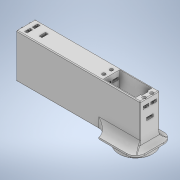
# Autodesk Inventor part: мотор_плеча_2.1-локтя_1_v2_увелич
Saved by Autodesk Inventor 2022 (Build 260153000, 153)
## iProperties
Created: 2022-12-03
Part Number: мотор_плеча_2.1-локтя_1_v2_увелич
Material: Типовые
Document SubType Name: Modeling
Designer: Папа
Density: 1 g/cm^3
Appearance: По умолчанию
Author: Папа
Autodesk Inventor part; units mm, degrees
(part 1 of 2)
ref_plane "YZ Plane" through (0, 0, 0) normal (1, 0, 0) x (0, 1, 0)
ref_plane "XZ Plane" through (0, 0, 0) normal (0, 1, 0) x (-1, 0, 0)
ref_plane "XY Plane" through (0, 0, 0) normal (0, 0, 1) x (1, 0, 0)
sketch "Эскиз1" plane through (0, 0, 0) normal (0, 1, 0) x (-1, 0, 0)
  line L0 (0, 0) -> (-59.05, 0)
  line L1 (-59.05, 0) -> (-59.05, -29.25)
  line L2 (-59.05, -29.25) -> (0, -29.25)
  line L3 (0, -29.25) -> (0, 0)
  line L4 (-74.05, 3) -> (15, 3)
  line L5 (15, 3) -> (15, -32.25)
  line L6 (15, -32.25) -> (-74.05, -32.25)
  line L7 (-74.05, -32.25) -> (-74.05, 3)
  line L8 (-74.05, 3) -> (15, -32.25) construction
  line L9 (15, 3) -> (-74.05, -32.25) construction
  line L10 (0, -29.25) -> (-59.05, 0) construction
  line L11 (0, 0) -> (-59.05, -29.25) construction
  line L12 (15, 0) -> (-74.05, 0)
  point P0 (-29.525, -14.625)
  point P1 (-29.525, -14.625)
  point P2 (-59.05, 0)
  point P3 (-59.05, 0)
  point P4 (0, 0)
  dimension "d0" = 29.25
  dimension "d1" = 59.05
  dimension "d2" = 15
  dimension "d3" = 3
  constraints: 26 end point, 4 midpoint, 4 parallel, 3 point on line, 2 horizontal, 2 perpendicular, 1 collinear
  measures "d0" distance of L2.end L0.start
  measures "d1" distance of L1.end L2.end
  measures "d2" distance between parallel lines of L3 L5
  measures "d3" distance between parallel lines of L6 L2
extrude "Выдавливание1" add sketch "Эскиз1" along normal blind 41 contours L12 L5 L6 L7 L1 L2 L3
sketch "Эскиз2" plane through (0, 0, 0) normal (0, -1, 0) x (1, 0, 0)
  line L0 (74.05, 0) -> (74.05, -32.25) projected
  line L1 (-15, -32.25) -> (-15, 0) projected
  line L2 (74.05, 0) -> (-15, 0)
  line L3 (-15, 0) -> (-15, -32.25)
  line L4 (-15, -32.25) -> (74.05, -32.25)
  line L5 (74.05, -32.25) -> (74.05, 0)
  point P0 (0, 0)
  constraints: 8 end point, 2 parallel, 1 horizontal, 1 perpendicular
extrude "Выдавливание2" add sketch "Эскиз2" along normal blind 3
sketch "Эскиз3" plane through (0, 41, 0) normal (0, 1, 0) x (1, 0, 0)
  circle A0 centre (-4.475, 5.225) radius 2.1
  circle A1 centre (-4.475, 24.225) radius 2.1
  circle A2 centre (63.525, 24.225) radius 2.1
  circle A3 centre (63.525, 5.225) radius 2.1
  line L0 (59.05, 29.25) -> (59.05, 0) construction
  line L1 (0, 0) -> (0, 29.25) construction
  line L2 (59.05, 29.25) -> (0, 29.25) construction
  line L3 (0, 29.25) -> (0, 0.2) construction
  line L4 (0, 0.2) -> (59.05, 0.2) construction
  line L5 (59.05, 0.2) -> (59.05, 29.25) construction
  line L6 (0, 0) -> (59.05, 0) construction
  line L7 (59.05, 0) -> (59.05, 0.2) construction
  line L8 (59.05, 0.2) -> (0, 0.2) construction
  line L9 (0, 0.2) -> (0, 0) construction
  line L10 (0, 0.2) -> (59.05, 29.25) construction
  line L11 (59.05, 0.2) -> (0, 29.25) construction
  line L12 (-4.475, 5.225) -> (63.525, 5.225) construction
  line L13 (63.525, 5.225) -> (63.525, 24.225) construction
  line L14 (63.525, 24.225) -> (-4.475, 24.225) construction
  line L15 (-4.475, 24.225) -> (-4.475, 5.225) construction
  line L16 (-4.475, 5.225) -> (63.525, 24.225) construction
  line L17 (-4.475, 24.225) -> (63.525, 5.225) construction
  point P0 (29.525, 14.725)
  dimension "d8" = 4.2
  dimension "d70" = 0.2
  dimension "d72" = 19
  dimension "d73" = 68
  constraints: 32 end point, 6 parallel, 4 centre point, 3 equal radius, 3 horizontal, 3 perpendicular, 2 coincident, 2 midpoint, 1 point on line
  measures "d8" diameter of A0
  measures "d70" distance between parallel lines of L4 L6
  measures "d72" distance of L13.end A3.centre
  measures "d73" distance of L13.end L14.end
extrude "Выдавливание3" cut sketch "Эскиз3" against normal blind 20
ref_plane "РабПлоскость1" through (0, 31, 0) normal (0, 1, 0) x (1, 0, 0)
sketch "Эскиз4" plane through (0, 31, 0) normal (0, 1, 0) x (1, 0, 0)
  circle A0 centre (63.525, 24.225) radius 2.1 projected
  line L0 (65.589, 27.8) -> (67.6531, 24.225)
  line L1 (67.6531, 24.225) -> (65.589, 20.65)
  line L2 (65.589, 20.65) -> (61.461, 20.65)
  line L3 (61.461, 20.65) -> (59.3969, 24.225)
  line L4 (59.3969, 24.225) -> (61.461, 27.8)
  line L5 (61.461, 27.8) -> (65.589, 27.8)
  circle A1 centre (-4.475, 24.225) radius 2.1 construction
  circle A2 centre (63.525, 5.225) radius 2.1 projected
  line L6 (-4.475, 24.225) -> (63.525, 24.225) construction
  line L7 (63.525, 24.225) -> (63.525, 5.225) construction
  line L8 (63.525, 5.225) -> (-4.475, 5.225) construction
  line L9 (-4.475, 5.225) -> (-4.475, 24.225) construction
  line L10 (-2.411, 27.8) -> (-0.3469, 24.225)
  line L11 (-0.3469, 24.225) -> (-2.411, 20.65)
  line L12 (-2.411, 20.65) -> (-6.539, 20.65)
  line L13 (-6.539, 20.65) -> (-8.6031, 24.225)
  line L14 (-8.6031, 24.225) -> (-6.539, 27.8)
  line L15 (-6.539, 27.8) -> (-2.411, 27.8)
  line L16 (65.589, 8.8) -> (67.6531, 5.225)
  line L17 (67.6531, 5.225) -> (65.589, 1.65)
  line L18 (65.589, 1.65) -> (61.461, 1.65)
  line L19 (61.461, 1.65) -> (59.3969, 5.225)
  line L20 (59.3969, 5.225) -> (61.461, 8.8)
  line L21 (61.461, 8.8) -> (65.589, 8.8)
  line L22 (-2.411, 8.8) -> (-0.3469, 5.225)
  line L23 (-0.3469, 5.225) -> (-2.411, 1.65)
  line L24 (-2.411, 1.65) -> (-6.539, 1.65)
  line L25 (-6.539, 1.65) -> (-8.6031, 5.225)
  line L26 (-8.6031, 5.225) -> (-6.539, 8.8)
  line L27 (-6.539, 8.8) -> (-2.411, 8.8)
  line L28 (65.589, 27.8) -> (74.05, 27.8)
  line L29 (74.05, 32.25) -> (74.05, 0) projected
  line L30 (65.589, 20.65) -> (74.05, 20.65)
  line L31 (29.525, 5.225) -> (29.525, 29.25) construction
  line L32 (0, 29.25) -> (59.05, 29.25) construction
  line L33 (0, 0) -> (0, 29.25) projected
  line L34 (0, 14.625) -> (59.05, 14.625) construction
  line L35 (59.05, 29.25) -> (59.05, 0) projected
  line L36 (59.05, 14.625) -> (0, 14.625) construction
  line L37 (-15, 27.8) -> (-15, 20.65)
  line L38 (-15, 0) -> (-15, 32.25) projected
  line L39 (65.589, 8.8) -> (74.05, 8.8)
  line L40 (65.589, 1.65) -> (74.05, 1.65)
  line L41 (74.05, 1.65) -> (74.05, 8.8)
  line L42 (-2.411, 27.8) -> (0, 27.8)
  line L43 (-2.411, 20.65) -> (0, 20.65)
  line L44 (0, 20.65) -> (0, 27.8)
  line L45 (-2.411, 8.8) -> (0, 8.8)
  line L46 (-2.411, 1.65) -> (0, 1.65)
  line L47 (0, 8.8) -> (0, 1.65)
  point P0 (-4.475, 24.225)
  point P1 (-4.475, 24.225)
  point P2 (63.525, 5.225)
  point P3 (63.525, 5.225)
  point P4 (-4.475, 5.225)
  point P5 (-4.475, 5.225)
  point P6 (-15, 1.45)
  point P7 (-15, 8.6)
  dimension "d14" = 7.15
  dimension "d17" = 68
  dimension "d20" = 19
  constraints: 86 end point, 8 point on line, 7 perpendicular, 6 symmetric about line, 4 collinear, 4 horizontal, 4 midpoint, 3 parallel, 1 coincident, 1 vertical, 55 other
  measures "d14" distance between parallel lines of L1 L4
  measures "d17" distance of point (63.525, 24.225) point (-4.475, 24.225)
  measures "d20" distance of point (63.525, 24.225) point (63.525, 5.225)
extrude "Выдавливание4" cut sketch "Эскиз4" against normal blind 3.25 contours A0 | L28 L29 L30 L1 L0 | L0 L1 L2 L3 L4 L5 | A2 | L42 L33 L43 L11 L10 | L10 L11 L12 L13 L14 L15 | L39 L29 L40 L17 L16 | L16 L17 L18 L19 L20 L21 | L45 L33 L46 L23 L22 | L22 L23 L24 L25 L26 L27
ref_plane "РабПлоскость2" through (0, 19, 0) normal (0, -1, 0) x (1, 0, 0)
ref_plane "РабПлоскость3" through (29.525, 41, -32.25) normal (-1, 0, 0) x (0, 0, 1)
ref_plane "РабПлоскость5" through (74.05, 41, 0) normal (0, -1, 0) x (-1, 0, 0)
sketch "Эскиз10" plane through (0, 41, 0) normal (0, 1, 0) x (1, 0, 0)
  line L0 (59.05, 0) -> (74.05, 0) projected
  line L1 (74.05, 32.25) -> (-15, 32.25) projected
  line L2 (74.05, 0) -> (-15, 0)
  line L3 (-15, 0) -> (-15, 32.25)
  line L4 (-15, 32.25) -> (74.05, 32.25)
  line L5 (74.05, 32.25) -> (74.05, 0)
  line L6 (0, 0) -> (0, 29.25) projected
  line L7 (59.05, 29.25) -> (59.05, 0) projected
  line L8 (0, 29.25) -> (59.05, 29.25)
  line L9 (59.05, 29.25) -> (59.05, 0)
  line L10 (59.05, 0) -> (0, 0)
  line L11 (0, 0) -> (0, 29.25)
  circle A0 centre (63.525, 24.225) radius 2.1 projected
  circle A1 centre (63.525, 24.225) radius 2.05
  circle A2 centre (63.525, 5.225) radius 2.05
  circle A3 centre (-4.475, 5.225) radius 2.1 projected
  circle A4 centre (-4.475, 5.225) radius 2.05
  circle A5 centre (-4.475, 24.225) radius 2.05
  circle A6 centre (-4.475, 24.225) radius 2.1 projected
  circle A7 centre (63.525, 5.225) radius 2.1 projected
  point P0 (74.05, 32.25)
  constraints: 16 end point, 6 coincident, 4 centre point, 4 parallel, 2 horizontal, 2 perpendicular
extrude "Выдавливание10" add sketch "Эскиз10" along normal blind 7 contours L7 L8 L6 L2 L3 L1 L5 L0 | A6 | A7
sketch "Эскиз11" plane through (74.05, 41, 0) normal (0, -1, 0) x (-1, 0, 0)
  line L0 (15, 29.25) -> (15, 0) projected
  line L1 (15, 0) -> (6.9, 0)
  line L2 (6.9, 0) -> (6.9, 29.05)
  line L3 (6.9, 29.05) -> (15, 29.05)
  line L4 (15, 29.05) -> (15, 0)
  point P0 (74.05, 0)
  point P1 (15, 29.05)
  dimension "d61" = 8.1
  constraints: 8 end point, 2 parallel, 1 horizontal, 1 perpendicular
  measures "d61" distance between parallel lines of L0 L2
extrude "Выдавливание11" cut sketch "Эскиз11" against normal blind 4
fillet "Сопряжение8" radius 1.95 1 edges at (67.15, 43, -29.05)
sketch "Эскиз13" plane through (74.05, 45, 0) normal (0, -1, 0) x (1, 0, 0)
  line L0 (-15, -29.25) -> (-15, 0) projected
  line L1 (-74.05, -29.25) -> (-15, -29.25) projected
  line L2 (-15, 0) -> (-15, -29.25)
  line L3 (-20, -13.625) -> (-10, -13.625)
  line L4 (-10, -13.625) -> (-10, -15.625)
  line L5 (-10, -15.625) -> (-20, -15.625)
  line L6 (-20, -15.625) -> (-20, -13.625)
  line L7 (-20, -13.625) -> (-10, -15.625) construction
  line L8 (-10, -13.625) -> (-20, -15.625) construction
  arc A0 (-11, -15.625) -> (-11, -13.625) centre (-11, -14.625) ccw
  line L9 (-10, -14.625) -> (-15, -14.625)
  line L10 (-15, -14.625) -> (-15, 0)
  line L11 (-15, 0) -> (-10, 0)
  line L12 (-10, 0) -> (-10, -14.625)
  point P0 (-74.05, 0)
  point P1 (-15, -13.625)
  dimension "d65" = 10
  dimension "d66" = 2
  constraints: 22 end point, 4 parallel, 3 midpoint, 3 point on circle, 3 tangent, 2 horizontal, 2 perpendicular, 2 point on line, 1 centre point, 1 vertical
  measures "d65" distance of L4.end L5.end
  measures "d66" distance of L3.end L4.end
extrude "Выдавливание12" cut sketch "Эскиз13" against normal blind 1.5
fillet "Сопряжение9" radius 1 1 edges at (64.05, 45.75, -15.625)
mirror "Зеркальное отражение2" about plane through (29.525, 41, -32.25) normal (-1, 0, 0) of "Выдавливание11", "Выдавливание12", "Сопряжение9"
sketch "Эскиз15" plane through (0, 48, 0) normal (0, 1, 0) x (1, 0, 0)
  arc A0 (42.1128, 0.625) -> (42.1128, 28.725) centre (44.775, 14.675) ccw
  line L0 (42.1128, 28.725) -> (10.5328, 28.725)
  line L1 (10.5328, 0.625) -> (42.1128, 0.625)
  arc A1 (10.5328, 20.7) -> (10.5328, 8.65) centre (10.5328, 14.675) ccw
  line L2 (10.5328, 28.725) -> (10.5328, 20.7)
  line L3 (10.5328, 8.65) -> (10.5328, 0.625)
  line L4 (-7.975, 29.225) -> (67.025, 29.225)
  line L5 (67.025, 29.225) -> (67.025, 0.125)
  line L6 (67.025, 0.125) -> (-7.975, 0.125)
  line L7 (-7.975, 0.125) -> (-7.975, 29.225)
  line L8 (-7.975, 29.225) -> (67.025, 0.125) construction
  line L9 (67.025, 29.225) -> (-7.975, 0.125) construction
  line L10 (59.075, 14.675) -> (67.025, 14.675)
  line L11 (10.5328, 20.7) -> (10.5328, 8.65) construction
  line L12 (67.025, 0.125) -> (-7.975, 0.125)
  line L13 (-7.975, 0.125) -> (-7.975, -2.875)
  line L14 (-7.975, -2.875) -> (67.025, -2.875)
  line L15 (67.025, -2.875) -> (67.025, 0.125)
  circle A2 centre (63.525, 24.225) radius 2.05
  circle A3 centre (63.525, 24.225) radius 2.1 projected
  circle A4 centre (-4.475, 24.225) radius 2.1 projected
  circle A5 centre (-4.475, 24.225) radius 2.1
  circle A6 centre (-4.475, 5.225) radius 2.1 projected
  circle A7 centre (-4.475, 5.225) radius 2.1
  circle A8 centre (63.525, 5.225) radius 2.05 projected
  circle A9 centre (63.525, 5.225) radius 2.05
  line L16 (4.5078, 14.675) -> (4.5078, 0)
  line L17 (59.05, 0) -> (0, 0) projected
  line L18 (29.525, 14.675) -> (29.525, 0)
  line L19 (74.05, 32.25) -> (-15, 32.25) projected
  line L20 (-15, 32.25) -> (29.525, 32.25)
  line L21 (29.525, 32.25) -> (29.525, 0)
  line L22 (29.525, 0) -> (-15, 0)
  line L23 (-15, 0) -> (-15, 32.25)
  point P0 (-52.75, -14.55)
  point P1 (29.525, 32.25)
  point P2 (-7.975, 0)
  point P3 (-7.975, 0.125)
  point P4 (4.5078, 0.125)
  point P5 (29.525, 28.725)
  dimension "d75" = 28.6
  dimension "d76" = 12.05
  dimension "d77" = 31.58
  dimension "d79" = 29.1
  dimension "d80" = 75
  dimension "d81" = 3
  dimension "d82" = 22.25
  dimension "d83" = 3.5
  dimension "d84" = 5
  dimension "d85" = 4.1
  dimension "d86" = 7.95
  dimension "d87" = 28.1
  constraints: 44 end point, 8 parallel, 6 centre point, 6 coincident, 6 point on circle, 5 horizontal, 5 perpendicular, 4 collinear, 4 midpoint, 1 point on line, 1 vertical
  measures "d75" diameter of A0
  measures "d76" diameter of A1
  measures "d77" distance of L1.start L1.end
  measures "d79" distance between parallel lines of L4 L6
  measures "d80" distance of L5.end L6.end
  measures "d81" distance of L14.end L5.end
  measures "d82" distance from line of L5 point (44.775, 14.675)
  measures "d83" distance from line of L5 A2.centre
  measures "d84" distance from line of L4 A2.centre
  measures "d85" diameter of A2
  measures "d86" distance of L10.start L10.end
  measures "d87" distance between parallel lines of L1 L0
extrude "Выдавливание13" add sketch "Эскиз15" along normal blind 4 contours L0 L2 A1 L16 L6 L7 L4 L21 | L16 L17 L22 L13 L6 | L4 L7 L13 L22 L23 L19 L21
sketch "Эскиз17" plane through (0, -3, 0) normal (0, -1, 0) x (1, 0, 0)
  circle A0 centre (63.525, -5.225) radius 2.05 projected
  circle A1 centre (63.525, -24.225) radius 2.1 projected
  line L0 (63.525, -5.225) -> (63.525, -24.225) construction
  line L1 (63.525, -14.725) -> (44.775, -14.725) construction
  circle A2 centre (44.775, -14.725) radius 18.9
  circle A3 centre (44.775, -14.725) radius 20.9
  point P0 (0, 0)
  dimension "d92" = 18.75
  dimension "d93" = 37.8
  dimension "d94" = 2
  constraints: 4 end point, 2 centre point, 2 coincident, 1 horizontal, 1 midpoint, 1 vertical
  measures "d92" distance of L1.start L1.end
  measures "d93" diameter of A2
  measures "d94" radial gap between concentric circles of A3 A2
extrude "Выдавливание15" add sketch "Эскиз17" along normal blind 6 contours A3 A0 | A0 A3 A1 | A1 A3 picked at (62.8379, -5.5731) picked at (62.8227, -23.8692)
sketch "Эскиз18" plane through (44.775, -9, -14.725) normal (0, -1, 0) x (1, 0, 0)
  circle A0 centre (0, 0) radius 18.9 projected
  circle A1 centre (-18.9, 0) radius 0.25
  line L0 (0, 0) -> (-17.8021, 0) construction
  point P0 (-44.775, 14.725)
  dimension "d99" = 0.5
  constraints: 2 end point, 1 centre point, 1 horizontal, 1 horizontal alignment, 1 other
  measures "d99" diameter of A1
extrude "Выдавливание16" add sketch "Эскиз18" against normal up to surface (6 mm away) contours A1 A0 | A0 A1 picked at (-18.8165, 0) picked at (-18.9826, -0.0101)
fillet "Сопряжение12" radius 0.7 2 edges at (25.8767, -6, -14.475) (25.8767, -6, -14.975)
pattern_circular "Круговой массив1" count 12 over 360 about axis through (44.775, -3, -14.725) along (0, -1, 0) of "Выдавливание16", "Сопряжение12"
fillet "Сопряжение14" radius 1.5 2 edges at (74.05, 22.5, 0) (74.05, 22.5, -32.25)
sketch "Эскиз27" plane through (-15, -3, -32.25) normal (-1, 0, 0) x (0, 0, 1)
  line L0 (32.25, 0) -> (32.25, 55) projected
  line L1 (0, 55) -> (32.25, 55) projected
  line L2 (0, 0) -> (0, 55) projected
  line L3 (32.25, 0) -> (0, 0) projected
  line L4 (0, 55) -> (32.25, 55) projected
  line L5 (16.125, 55) -> (16.125, 28) construction
  line L6 (28.125, 56) -> (4.125, 56)
  line L7 (4.125, 56) -> (4.125, 0)
  line L8 (4.125, 0) -> (28.125, 0)
  line L9 (28.125, 0) -> (28.125, 56)
  line L10 (28.125, 56) -> (4.125, 0) construction
  line L11 (4.125, 56) -> (28.125, 0) construction
  point P0 (32.25, 3)
  point P1 (28.125, 55)
  point P2 (4.125, 55)
  dimension "d148" = 27
  dimension "d149" = 24
  constraints: 14 end point, 3 midpoint, 2 parallel, 1 horizontal, 1 perpendicular, 1 point on line, 1 vertical
  measures "d148" distance of L5.start L5.end
  measures "d149" distance between parallel lines of L7 L9
extrude "Выдавливание24" add sketch "Эскиз27" along normal blind 50 contours L3 L7 L1 L9
sketch "Эскиз28" plane through (-65, -3, -32.25) normal (-1, 0, 0) x (0, 0, 1)
  line L0 (28.125, 55) -> (4.125, 55) projected
  line L1 (4.125, 55) -> (4.125, 0) projected
  line L2 (4.125, 0) -> (28.125, 0) projected
  line L3 (28.125, 0) -> (28.125, 55) projected
  line L4 (4.125, 0) -> (4.125, 55) projected
  line L5 (28.125, 0) -> (4.125, 55) construction
  line L6 (26.175, 47.55) -> (6.075, 47.55)
  line L7 (6.075, 47.55) -> (6.075, 7.45)
  line L8 (6.075, 7.45) -> (26.175, 7.45)
  line L9 (26.175, 7.45) -> (26.175, 47.55)
  line L10 (26.175, 47.55) -> (6.075, 7.45) construction
  line L11 (6.075, 47.55) -> (26.175, 7.45) construction
  point P0 (32.25, 3)
  point P1 (16.125, 27.5)
  dimension "d152" = 40.1
  dimension "d153" = 20.1
  constraints: 14 end point, 3 midpoint, 2 parallel, 1 horizontal, 1 perpendicular
  measures "d152" distance between parallel lines of L6 L8
  measures "d153" distance between parallel lines of L9 L7
extrude "Выдавливание25" add sketch "Эскиз28" along normal blind 27.5
sketch "Эскиз29" plane through (-92.5, -3, -32.25) normal (-1, 0, 0) x (0, 0, 1)
  line L0 (4.125, 55) -> (4.125, 0) construction
  line L1 (4.125, 0) -> (28.125, 0) construction
  line L2 (28.125, 0) -> (28.125, 55) construction
  line L3 (28.125, 55) -> (4.125, 55) construction
  line L4 (26.175, 47.55) -> (26.175, 7.45) construction
  line L5 (26.175, 7.45) -> (6.075, 7.45) construction
  line L6 (6.075, 7.45) -> (6.075, 47.55) construction
  line L7 (6.075, 47.55) -> (26.175, 47.55) construction
  line L8 (32.25, 0) -> (28.125, 0) construction
  line L9 (28.125, 0) -> (4.125, 55) construction
  line L10 (20.875, 52.7) -> (11.375, 52.7) construction
  line L11 (11.375, 52.7) -> (11.375, 2.3) construction
  line L12 (11.375, 2.3) -> (20.875, 2.3) construction
  line L13 (20.875, 2.3) -> (20.875, 52.7) construction
  line L14 (20.875, 52.7) -> (11.375, 2.3) construction
  line L15 (11.375, 52.7) -> (20.875, 2.3) construction
  circle A0 centre (11.375, 52.7) radius 2.05
  circle A1 centre (20.875, 52.7) radius 2.05
  circle A2 centre (20.875, 2.3) radius 2.05
  circle A3 centre (11.375, 2.3) radius 2.05
  point P0 (32.25, 3)
  point P1 (16.125, 27.5)
  dimension "d156" = 9.5
  dimension "d157" = 50.4
  dimension "d158" = 4.1
  constraints: 14 end point, 4 centre point, 4 coincident, 3 equal radius, 3 midpoint, 2 parallel, 1 horizontal, 1 perpendicular
  measures "d156" distance of L11.end L12.end
  measures "d157" distance of L10.end L11.end
  measures "d158" diameter of A0
extrude "Выдавливание26" cut sketch "Эскиз29" against normal blind 15
ref_plane "РабПлоскость8" through (-82.5, -3, -32.25) normal (-1, 0, 0) x (0, 0, 1)
sketch "Эскиз30" plane through (-82.5, -3, -32.25) normal (-1, 0, 0) x (0, 0, 1)
  circle A0 centre (20.875, 2.3) radius 2.05 construction
  circle A1 centre (11.375, 2.3) radius 2.05 construction
  circle A2 centre (11.375, 52.7) radius 2.05 construction
  line L0 (20.875, 2.3) -> (11.375, 2.3) construction
  line L1 (32.25, 3) -> (3, 3) construction
  line L2 (11.375, 2.3) -> (11.375, 52.7) construction
  line L3 (11.375, -1.7415) -> (7.875, 0.2793)
  line L4 (7.875, 0.2793) -> (7.875, 4.3207)
  line L5 (7.875, 4.3207) -> (11.375, 6.3415)
  line L6 (11.375, 6.3415) -> (14.875, 4.3207)
  line L7 (14.875, 4.3207) -> (14.875, 0.2793)
  line L8 (14.875, 0.2793) -> (11.375, -1.7415)
  line L9 (20.875, -1.7415) -> (17.375, 0.2793)
  line L10 (17.375, 0.2793) -> (17.375, 4.3207)
  line L11 (17.375, 4.3207) -> (20.875, 6.3415)
  line L12 (20.875, 6.3415) -> (24.375, 4.3207)
  line L13 (24.375, 4.3207) -> (24.375, 0.2793)
  line L14 (24.375, 0.2793) -> (20.875, -1.7415)
  line L15 (11.375, 48.6585) -> (7.875, 50.6793)
  line L16 (7.875, 50.6793) -> (7.875, 54.7207)
  line L17 (7.875, 54.7207) -> (11.375, 56.7415)
  line L18 (11.375, 56.7415) -> (14.875, 54.7207)
  line L19 (14.875, 54.7207) -> (14.875, 50.6793)
  line L20 (14.875, 50.6793) -> (11.375, 48.6585)
  line L21 (20.875, 48.6585) -> (17.375, 50.6793)
  line L22 (17.375, 50.6793) -> (17.375, 54.7207)
  line L23 (17.375, 54.7207) -> (20.875, 56.7415)
  line L24 (20.875, 56.7415) -> (24.375, 54.7207)
  line L25 (24.375, 54.7207) -> (24.375, 50.6793)
  line L26 (24.375, 50.6793) -> (20.875, 48.6585)
  line L27 (24.375, 54.7207) -> (24.375, 58.7622)
  line L28 (24.375, 58.7622) -> (17.375, 58.7622)
  line L29 (17.375, 58.7622) -> (17.375, 54.7207)
  line L30 (7.875, 58.7622) -> (7.875, 54.7207)
  line L31 (14.875, 58.7622) -> (7.875, 58.7622)
  line L32 (14.875, 54.7207) -> (14.875, 58.7622)
  line L33 (17.375, 109.1622) -> (17.375, 105.1207)
  line L34 (24.375, 109.1622) -> (17.375, 109.1622)
  line L35 (24.375, 105.1207) -> (24.375, 109.1622)
  line L36 (7.875, 109.1622) -> (7.875, 105.1207)
  line L37 (14.875, 109.1622) -> (7.875, 109.1622)
  line L38 (14.875, 105.1207) -> (14.875, 109.1622)
  line L39 (26.175, 47.55) -> (6.075, 47.55) projected
  line L40 (6.075, 47.55) -> (6.075, 7.45) projected
  line L41 (6.075, 7.45) -> (26.175, 7.45) projected
  line L42 (26.175, 7.45) -> (26.175, 47.55) projected
  line L43 (26.175, 7.45) -> (6.075, 47.55) construction
  line L44 (6.075, 7.45) -> (26.175, 47.55) construction
  line L45 (16.125, 27.5) -> (26.175, 27.5) construction
  line L46 (7.875, -3.7622) -> (14.875, -3.7622)
  line L47 (17.375, -3.7622) -> (24.375, -3.7622)
  line L48 (24.375, -3.7622) -> (24.375, 0.2793)
  line L49 (17.375, 0.2793) -> (17.375, -3.7622)
  line L50 (14.875, -3.7622) -> (14.875, 0.2793)
  line L51 (7.875, 0.2793) -> (7.875, -3.7622)
  line L52 (7.875, 54.7207) -> (14.875, 54.7207)
  line L53 (11.55, 55) -> (3.525, 55) projected
  line L54 (7.875, 0.2793) -> (14.875, 0.2793)
  line L55 (32.25, 0) -> (0, 0) projected
  line L56 (17.375, 0.2793) -> (24.375, 0.2793)
  line L57 (18.1794, 0) -> (26.4026, 0) projected
  point P0 (19.8939, 0)
  point P1 (21.8561, 0)
  point P2 (10.3939, 0)
  point P3 (12.3561, 0)
  point P4 (12.3561, 54)
  point P5 (10.3939, 54)
  point P6 (20.875, 2.3)
  point P7 (11.375, 52.7)
  point P8 (20.875, 52.7)
  point P9 (20.875, -1.7415)
  point P10 (11.375, -1.7415)
  point P11 (17.375, 0.2793)
  point P12 (7.875, 0.2793)
  point P13 (7.875, 54.7207)
  dimension "d162" = 7
  dimension "d165" = 9.5
  dimension "d168" = 50.4
  dimension "d214" = 9.5
  dimension "d217" = 50.4
  dimension "d222" = 360
  constraints: 100 end point, 4 parallel, 4 vertical, 3 perpendicular, 2 collinear, 2 horizontal, 2 midpoint, 1 coincident, 107 other
  measures "d162" distance between parallel lines of L7 L4
  measures "d165" distance of point (11.375, 2.3) point (20.875, 2.3)
  measures "d168" distance of point (11.375, 2.3) point (11.375, 52.7)
  measures "d214" distance of L28.end L30.start
  measures "d217" distance of L28.end L33.start
extrude "Выдавливание27" cut sketch "Эскиз30" along normal blind 3.3 contours L8 L55 L50 L46 L51 L3 | L3 L55 L8 | L55 L51 L3 | L3 L54 L8 L55 | L8 L50 L55 | L4 L5 L6 L7 L54 | L14 L55 L48 L47 L49 L9 | L9 L55 L14 | L55 L49 L9 | L9 L56 L14 L55 | L14 L48 L55 | L10 L11 L12 L13 L56 | L15 L16 L52 L19 L20 | L30 L53 L17 | L17 L18 L52 | L18 L17 L53 L30 L31 L32 | L21 L22 L23 L24 L25 L26 | L29 L28 L27 L24 L23
sketch "Эскиз31" plane through (0, 52, 0) normal (0, 1, 0) x (1, 0, 0)
  line L0 (-85.8, 17.375) -> (-85.8, 24.375) construction
  line L1 (-92.5, 4.125) -> (-92.5, 28.125) construction
  line L2 (-85.8, 7.875) -> (-85.8, 14.875) construction
  line L3 (-82.5, 24.375) -> (-82.5, 17.375) construction
  line L4 (-82.5, 14.875) -> (-82.5, 7.875) construction
  line L5 (-15, 4.125) -> (-92.5, 4.125) construction
  line L6 (-15, 4.125) -> (-15, 0) construction
  line L7 (-15, 0) -> (4.5078, 0) construction
  line L8 (4.5078, 0) -> (4.5078, 14.675) construction
  arc A0 (10.5328, 20.7) -> (4.5078, 14.675) centre (10.5328, 14.675) ccw construction
  line L9 (10.5328, 20.7) -> (10.5328, 28.725) construction
  line L10 (10.5328, 28.725) -> (29.525, 28.725) construction
  line L11 (29.525, 28.725) -> (29.525, 32.25) construction
  line L12 (29.525, 32.25) -> (-15, 32.25) construction
  line L13 (-15, 32.25) -> (-15, 28.125) construction
  line L14 (-15, 28.125) -> (-92.5, 28.125) construction
  circle A1 centre (-4.475, 5.225) radius 2.1 construction
  circle A2 centre (-4.475, 24.225) radius 2.1 construction
  line L15 (-15, 28.125) -> (-15, 32.25) construction
  line L16 (-92.5, 10.3939) -> (-92.5, 4.125) construction
  line L17 (-15, 28.125) -> (-92.5, 28.125) construction
  line L18 (-92.5, 28.125) -> (-92.5, 4.125) construction
  line L19 (-92.5, 4.125) -> (-15, 4.125) construction
  line L20 (-15, 4.125) -> (-15, 28.125) construction
  line L21 (-15, 16.125) -> (-70, 16.125) construction
  line L22 (-70, 16.125) -> (-70, 28.125) construction
  line L23 (-15, 28.125) -> (-92.5, 28.125) construction
  line L24 (-71.75, 20.125) -> (-68.25, 20.125)
  line L25 (-68.25, 20.125) -> (-68.25, 12.125)
  line L26 (-68.25, 12.125) -> (-71.75, 12.125)
  line L27 (-71.75, 12.125) -> (-71.75, 20.125)
  line L28 (-71.75, 20.125) -> (-68.25, 12.125) construction
  line L29 (-68.25, 20.125) -> (-71.75, 12.125) construction
  line L30 (-82.5, 7.875) -> (-85.8, 7.875) projected
  line L31 (-85.8, 14.875) -> (-82.5, 14.875) projected
  line L32 (-82.5, 17.375) -> (-85.8, 17.375) projected
  line L33 (-85.8, 24.375) -> (-82.5, 24.375) projected
  dimension "d173" = 55
  dimension "d174" = 3.5
  dimension "d175" = 8
  constraints: 24 end point, 4 parallel, 3 horizontal, 3 midpoint, 3 perpendicular, 1 point on line
  measures "d173" distance of L21.start L21.end
  measures "d174" distance of L25.end L26.end
  measures "d175" distance of L26.end L24.start
extrude "Выдавливание28" cut sketch "Эскиз31" against normal blind 10
sketch "Эскиз32" plane through (-92.5, -3, -32.25) normal (-1, 0, 0) x (0, 0, 1)
  line L0 (20.125, 55) -> (12.125, 55) projected
  line L1 (6.075, 47.55) -> (26.175, 47.55) projected
  line L2 (12.125, 55) -> (12.125, 47.55)
  line L3 (12.125, 55) -> (12.125, 47.55) projected
  line L4 (20.125, 55) -> (20.125, 47.55)
  line L5 (20.125, 55) -> (20.125, 47.55) projected
  line L6 (12.125, 47.55) -> (20.125, 47.55)
  line L7 (20.125, 47.55) -> (20.125, 49.05)
  line L8 (20.125, 49.05) -> (12.125, 49.05)
  line L9 (12.125, 49.05) -> (12.125, 47.55)
  point P0 (32.25, 3)
  point P1 (12.625, 44)
  point P2 (19.625, 44)
  dimension "d178" = 1.5
  constraints: 12 end point, 2 parallel, 2 point on line, 1 horizontal, 1 perpendicular, 5 other
  measures "d178" distance between parallel lines of L1 L8
extrude "Выдавливание29" cut sketch "Эскиз32" against normal up to surface (24.25 mm away) contours L4 L1 L2 L8
sketch "Эскиз33" plane through (0, -3, 0) normal (0, -1, 0) x (1, 0, 0)
  arc A0 (29.9431, 0) -> (33.3871, -32.25) centre (44.775, -14.725) ccw construction
  circle A1 centre (44.775, -14.725) radius 20.9 construction
  line L0 (23.875, -35.625) -> (65.675, -35.625) construction
  line L1 (65.675, -35.625) -> (65.675, 6.175) construction
  line L2 (65.675, 6.175) -> (23.875, 6.175) construction
  line L3 (23.875, 6.175) -> (23.875, -35.625) construction
  line L4 (23.875, -35.625) -> (65.675, 6.175) construction
  line L5 (65.675, -35.625) -> (23.875, 6.175) construction
  line L6 (21.875, -37.625) -> (67.675, -37.625)
  line L7 (67.675, -37.625) -> (67.675, 8.175)
  line L8 (67.675, 8.175) -> (21.875, 8.175)
  line L9 (21.875, 8.175) -> (21.875, -37.625)
  line L10 (21.875, -37.625) -> (67.675, 8.175) construction
  line L11 (67.675, -37.625) -> (21.875, 8.175) construction
  line L12 (59.05, 0) -> (0, 0) projected
  line L13 (74.05, -1.5) -> (74.05, -30.75) projected
  line L14 (14.1054, 0) -> (86.1611, 0) construction
  line L15 (74.05, -27.8) -> (74.05, -20.65) projected
  line L16 (74.05, -26.45) -> (74.05, 10.0078) construction
  circle A2 centre (44.775, -14.725) radius 32.7697 construction
  line L17 (29.9431, 0) -> (-15, 0) projected
  line L18 (21.875, 0) -> (67.675, 0)
  line L19 (59.05, 0) -> (72.55, 0) projected
  line L20 (56.1629, -32.25) -> (72.55, -32.25) projected
  line L21 (67.675, -32.25) -> (21.875, -32.25)
  line L22 (-15, -32.25) -> (33.3871, -32.25) projected
  point P0 (21.875, 0)
  dimension "d182" = 2
  constraints: 32 end point, 11 point on line, 4 midpoint, 4 parallel, 4 perpendicular, 2 centre point, 2 coincident, 2 horizontal, 1 collinear, 1 point on circle, 1 tangent
  measures "d182" distance between parallel lines of L8 L2
extrude "Выдавливание30" add sketch "Эскиз33" against normal up to surface (3 mm away) contours L9 L21 L20 L7 L6 | L9 L8 L7 L18 L12
sketch "Эскиз34" plane through (74.05, -3, -30.75) normal (1, 0, 0) x (0, 0, -1)
  line L0 (37.7171, -24.9258) -> (-58.7983, -24.9258)
  line L1 (-58.7983, -24.9258) -> (-58.7983, 82.8579)
  line L2 (-58.7983, 82.8579) -> (37.7171, 82.8579)
  line L3 (37.7171, 82.8579) -> (37.7171, -24.9258)
  point P0 (-30.75, 3)
  constraints: 8 end point, 2 parallel, 1 horizontal, 1 perpendicular
extrude "Выдавливание31" cut sketch "Эскиз34" against normal blind 1.5
sketch "Эскиз35" plane through (59.05, 41, 0) normal (0, 0, 1) x (1, 0, 0)
  line L0 (0, -41) -> (0, 0) projected
  line L1 (0, -41) -> (0, -35.5)
  line L2 (0, -35.5) -> (1.2932, -35.5)
  line L3 (1.2932, -35.5) -> (1.2932, -32.5)
  line L4 (1.2932, -32.5) -> (0, -32.5)
  line L5 (0, -32.5) -> (0, -35.5)
  point P0 (-59.05, -41)
  point P1 (0, -32.5)
  dimension "d190" = 5.5
  dimension "d191" = 3
  constraints: 10 end point, 2 parallel, 1 horizontal, 1 perpendicular, 1 vertical
  measures "d190" distance of L0.start L1.end
  measures "d191" distance of L2.end L3.end
extrude "Выдавливание32" cut sketch "Эскиз35" against normal blind 18
sketch "Эскиз36" plane through (0, 48, 0) normal (0, 1, 0) x (1, 0, 0)
  circle A0 centre (63.525, 5.225) radius 2.1 projected
  circle A1 centre (63.525, 24.225) radius 2.1 projected
  line L0 (63.525, 5.225) -> (63.525, 24.225)
  line L1 (63.525, 14.725) -> (61.1407, 16.0366)
  point P0 (0, 0)
  constraints: 4 end point, 1 midpoint, 1 vertical
sketch "Эскиз37" plane through (59.05, 41, -18) normal (0, 0, 1) x (1, 0, 0)
  line L0 (0, -32.5) -> (1.2932, -32.5) projected
  line L1 (1.2932, -32.5) -> (1.2932, -35.5) projected
  line L2 (1.2932, -35.5) -> (0, -35.5) projected
  line L3 (0, -41) -> (0, -35.5) projected
  line L4 (0, -41) -> (8.625, -41) projected
  line L5 (8.625, -41) -> (8.625, -44) projected
  line L6 (-37.175, -44) -> (-74.05, -44) projected
  line L7 (0, 7) -> (13.5, 7) projected
  line L8 (0, 5.5) -> (0, 7) projected
  line L9 (0, 5.5) -> (5, 5.5) projected
  line L10 (5, 5.5) -> (5, 4) projected
  line L11 (5, 4) -> (8.1, 4) projected
  line L12 (8.1, 4) -> (8.1, 0) projected
  line L13 (8.1, 0) -> (0, 0) projected
  line L14 (0, -32.5) -> (0, 0) projected
  line L15 (0, -35.5) -> (13.5, -35.5)
  line L16 (13.5, -35.5) -> (13.5, -32.5)
  line L17 (13.5, -32.5) -> (0, -32.5)
  line L18 (0, -32.5) -> (0, -35.5)
  line L19 (13.5, 7) -> (13.5, -44) projected
  line L20 (13.5, 7) -> (13.5, -44) projected
  line L21 (-37.175, -44) -> (-37.175, -41) projected
  line L22 (-37.175, -41) -> (-59.05, -41) projected
  line L23 (-59.05, -41) -> (-59.05, 0) projected
  line L24 (-59.05, 0) -> (-67.15, 0) projected
  line L25 (-67.15, 0) -> (-67.15, 4) projected
  line L26 (-67.15, 4) -> (-64.05, 4) projected
  line L27 (-64.05, 4) -> (-64.05, 5.5) projected
  line L28 (-64.05, 5.5) -> (-59.05, 5.5) projected
  line L29 (-59.05, 5.5) -> (-59.05, 7) projected
  line L30 (-59.05, 7) -> (-54.5422, 7) projected
  line L31 (-54.5422, 7) -> (-54.5422, 11) projected
  line L32 (-74.05, 11) -> (-54.5422, 11) projected
  line L33 (-74.05, -44) -> (-74.05, 11) projected
  line L34 (13.5, -44) -> (8.625, -44) projected
  constraints: 8 end point, 2 collinear, 2 parallel, 1 horizontal, 1 perpendicular
extrude "Выдавливание33" cut sketch "Эскиз37" along normal blind 6.55 contours L0 L1 L2 L18 | L17 L16 L15 L1
sketch "Эскиз38" plane through (72.55, -3, -30.75) normal (1, 0, 0) x (0, 0, -1)
  line L0 (-38.925, -6) -> (6.875, -6)
  line L1 (6.875, -6) -> (6.875, 55)
  line L2 (6.875, 55) -> (-38.925, 55)
  line L3 (-38.925, 55) -> (-38.925, -6)
  line L4 (-36.925, -6) -> (4.875, -6) projected
  line L5 (6.875, 0) -> (6.875, 3) projected
  line L6 (-38.925, 0) -> (-38.925, 3) projected
  line L7 (-30.75, 55) -> (-16.075, 55) projected
  point P0 (-30.75, 3)
  constraints: 8 end point, 4 collinear, 2 parallel, 1 horizontal, 1 perpendicular
extrude "Выдавливание34" cut sketch "Эскиз38" against normal up to surface (87.55 mm away)
sketch "Эскиз39" plane through (-15, -3, -4.125) normal (1, 0, 0) x (0, 0, -1)
  line L0 (24, 0) -> (0, 0) projected
  line L1 (0, 55) -> (24, 55) projected
  line L2 (0, 0) -> (24, 0)
  line L3 (24, 0) -> (24, 55)
  line L4 (24, 55) -> (0, 55)
  line L5 (0, 55) -> (0, 0)
  point P0 (-4.125, 3)
  constraints: 8 end point, 2 parallel, 1 horizontal, 1 perpendicular
extrude "Выдавливание35" add sketch "Эскиз39" along normal blind 77.5
sketch "Эскиз40" plane through (0, 52, 0) normal (0, 1, 0) x (1, 0, 0)
  line L0 (55.05, 6.075) -> (14.95, 6.075)
  line L1 (14.95, 6.075) -> (14.95, 26.175)
  line L2 (14.95, 26.175) -> (55.05, 26.175)
  line L3 (55.05, 26.175) -> (55.05, 6.075)
  line L4 (62.5, 28.125) -> (-92.5, 28.125) projected
  line L5 (62.5, 28.125) -> (62.5, 4.125) projected
  line L6 (-92.5, 4.125) -> (62.5, 4.125) projected
  line L7 (35, 26.175) -> (35, 28.125) construction
  line L8 (35, 6.075) -> (35, 4.125) construction
  point P0 (0, 0)
  dimension "d201" = 7.45
  dimension "d202" = 20.1
  dimension "d203" = 40.1
  constraints: 12 end point, 3 point on line, 2 midpoint, 2 parallel, 1 collinear, 1 horizontal, 1 perpendicular, 1 vertical
  measures "d201" distance between parallel lines of L5 L3
  measures "d202" distance between parallel lines of L0 L2
  measures "d203" distance between parallel lines of L1 L3
extrude "Выдавливание36" cut sketch "Эскиз40" against normal blind 27.5
sketch "Эскиз41" plane through (0, 52, 0) normal (0, 1, 0) x (1, 0, 0)
  line L0 (60.2, 11.375) -> (9.8, 11.375) construction
  line L1 (9.8, 11.375) -> (9.8, 20.875) construction
  line L2 (9.8, 20.875) -> (60.2, 20.875) construction
  line L3 (60.2, 20.875) -> (60.2, 11.375) construction
  line L4 (14.95, 6.075) -> (14.95, 26.175) construction
  line L5 (55.05, 26.175) -> (55.05, 6.075) construction
  line L6 (9.8, 20.875) -> (60.2, 11.375) construction
  line L7 (60.2, 20.875) -> (9.8, 11.375) construction
  line L8 (55.05, 26.175) -> (55.05, 6.075) construction
  line L9 (14.95, 26.175) -> (55.05, 26.175) construction
  line L10 (55.05, 6.075) -> (14.95, 26.175) construction
  line L11 (55.05, 6.075) -> (14.95, 6.075) construction
  line L12 (14.95, 6.075) -> (55.05, 26.175) construction
  circle A0 centre (60.2, 20.875) radius 2.05
  circle A1 centre (60.2, 11.375) radius 2.05
  circle A2 centre (9.8, 11.375) radius 2.05
  circle A3 centre (9.8, 20.875) radius 2.05
  point P0 (0, 0)
  point P1 (35, 16.125)
  dimension "d206" = 50.4
  dimension "d207" = 9.5
  dimension "d208" = 4.1
  constraints: 16 end point, 4 centre point, 4 coincident, 3 equal radius, 2 midpoint, 2 parallel, 1 horizontal, 1 perpendicular
  measures "d206" distance of L1.end L2.end
  measures "d207" distance of L0.end L1.end
  measures "d208" diameter of A0
extrude "Выдавливание37" cut sketch "Эскиз41" against normal blind 15
ref_plane "РабПлоскость9" through (0, 45.3, 0) normal (0, 1, 0) x (1, 0, 0)
sketch "Эскиз42" plane through (0, 45.3, 0) normal (0, 1, 0) x (1, 0, 0)
  circle A0 centre (9.8, 20.875) radius 2.05 projected
  circle A1 centre (9.8, 11.375) radius 2.05 projected
  circle A2 centre (60.2, 11.375) radius 2.05 projected
  circle A3 centre (60.2, 20.875) radius 2.05 projected
  line L0 (13.8415, 20.875) -> (11.8207, 17.375)
  line L1 (11.8207, 17.375) -> (7.7793, 17.375)
  line L2 (7.7793, 17.375) -> (5.7585, 20.875)
  line L3 (5.7585, 20.875) -> (7.7793, 24.375)
  line L4 (7.7793, 24.375) -> (11.8207, 24.375)
  line L5 (11.8207, 24.375) -> (13.8415, 20.875)
  line L6 (11.8207, 24.375) -> (14.95, 24.375)
  line L7 (14.95, 24.375) -> (14.95, 17.375)
  line L8 (14.95, 6.075) -> (14.95, 26.175) projected
  line L9 (11.8207, 17.375) -> (14.95, 17.375)
  line L10 (64.2415, 20.875) -> (62.2207, 17.375)
  line L11 (62.2207, 17.375) -> (58.1793, 17.375)
  line L12 (58.1793, 17.375) -> (56.1585, 20.875)
  line L13 (56.1585, 20.875) -> (58.1793, 24.375)
  line L14 (58.1793, 24.375) -> (62.2207, 24.375)
  line L15 (62.2207, 24.375) -> (64.2415, 20.875)
  line L16 (62.2207, 24.375) -> (65.35, 24.375)
  line L17 (65.35, 24.375) -> (65.35, 17.375)
  line L18 (62.2207, 17.375) -> (65.35, 17.375)
  line L19 (13.8415, 11.375) -> (11.8207, 7.875)
  line L20 (11.8207, 7.875) -> (7.7793, 7.875)
  line L21 (7.7793, 7.875) -> (5.7585, 11.375)
  line L22 (5.7585, 11.375) -> (7.7793, 14.875)
  line L23 (7.7793, 14.875) -> (11.8207, 14.875)
  line L24 (11.8207, 14.875) -> (13.8415, 11.375)
  line L25 (11.8207, 14.875) -> (14.95, 14.875)
  line L26 (14.95, 14.875) -> (14.95, 7.875)
  line L27 (11.8207, 7.875) -> (14.95, 7.875)
  line L28 (64.2415, 11.375) -> (62.2207, 7.875)
  line L29 (62.2207, 7.875) -> (58.1793, 7.875)
  line L30 (58.1793, 7.875) -> (56.1585, 11.375)
  line L31 (56.1585, 11.375) -> (58.1793, 14.875)
  line L32 (58.1793, 14.875) -> (62.2207, 14.875)
  line L33 (62.2207, 14.875) -> (64.2415, 11.375)
  line L34 (62.2207, 14.875) -> (65.35, 14.875)
  line L35 (65.35, 14.875) -> (65.35, 7.875)
  line L36 (62.2207, 7.875) -> (65.35, 7.875)
  point P0 (0, 0)
  point P1 (60.2, 20.875)
  point P2 (9.8, 11.375)
  point P3 (60.2, 11.375)
  dimension "d224" = 7
  dimension "d227" = 50.4
  dimension "d230" = 9.5
  constraints: 72 end point, 3 horizontal, 2 collinear, 2 perpendicular, 1 coincident, 1 point on line, 1 vertical, 65 other
  measures "d224" distance between parallel lines of L1 L4
  measures "d227" distance of point (9.8, 20.875) point (60.2, 20.875)
  measures "d230" distance of point (9.8, 20.875) point (9.8, 11.375)
extrude "Выдавливание38" cut sketch "Эскиз42" against normal blind 3.3 contours A0 | A1 | A2 | A3 | L5 L6 L7 L9 L0 | L0 L1 L2 L3 L4 L5 | L27 L19 L24 L25 L8 | L20 L21 L22 L23 L24 L19 | L15 L16 L17 L18 L10 | L10 L11 L12 L13 L14 L15 | L33 L34 L35 L36 L28 | L28 L29 L30 L31 L32 L33
sketch "Эскиз43" plane through (0, 52, 0) normal (0, 1, 0) x (1, 0, 0)
  line L0 (55.05, 26.175) -> (55.05, 6.075) projected
  line L1 (55.05, 12.125) -> (56.55, 12.125)
  line L2 (56.55, 12.125) -> (56.55, 20.125)
  line L3 (56.55, 20.125) -> (55.05, 20.125)
  line L4 (55.05, 20.125) -> (55.05, 12.125)
  line L5 (55.05, 26.175) -> (57.5417, 16.125) construction
  line L6 (57.5417, 16.125) -> (55.05, 6.075) construction
  point P0 (0, 0)
  dimension "d235" = 1.5
  dimension "d236" = 8
  constraints: 12 end point, 3 point on line, 2 parallel, 1 equal length, 1 horizontal, 1 perpendicular
  measures "d235" distance of L2.end L3.end
  measures "d236" distance of L1.end L2.end
extrude "Выдавливание39" cut sketch "Эскиз43" against normal blind 24.25
sketch "Эскиз44" plane through (56.55, 52, -20.125) normal (-1, 0, 0) x (0, 0, 1)
  line L0 (0, -24.25) -> (8, -24.25) projected
  line L1 (0, 0) -> (8, 0) projected
  line L2 (0, 0) -> (0, -24.25) projected
  line L3 (0, -24.25) -> (8, -24.25) projected
  line L4 (8, 0) -> (8, -24.25) projected
  line L5 (0, 0) -> (0, -24.25) projected
  line L6 (0, -20.75) -> (8, -20.75)
  line L7 (8, 0) -> (8, -24.25) projected
  point P0 (20.125, -52)
  dimension "d241" = 3.5
  constraints: 2 end point, 2 point on line, 1 horizontal
  measures "d241" distance between parallel lines of L6 L0
extrude "Выдавливание40" cut sketch "Эскиз44" against normal blind 24.25 contours L2 L6 L4 L0
sketch "Эскиз45" plane through (0, -3, 0) normal (0, -1, 0) x (1, 0, 0)
  circle A0 centre (45, -16.125) radius 18.65
  circle A1 centre (60.2, -20.875) radius 2.05 construction
  circle A2 centre (60.2, -20.875) radius 2.05 construction
  circle A3 centre (60.2, -11.375) radius 2.05 construction
  circle A4 centre (60.2, -11.375) radius 2.05 construction
  line L0 (60.2, -11.375) -> (60.2, -20.875) construction
  line L1 (60.2, -16.125) -> (45, -16.125) construction
  circle A5 centre (45, -16.125) radius 21.15
  point P0 (0, 0)
  dimension "d244" = 15.2
  dimension "d245" = 37.3
  dimension "d246" = 2.5
  constraints: 4 end point, 2 centre point, 2 coincident, 1 midpoint, 1 perpendicular, 1 vertical
  measures "d244" distance of L1.start L1.end
  measures "d245" diameter of A0
  measures "d246" radial gap between concentric circles of A0 A5
extrude "Выдавливание41" add sketch "Эскиз45" along normal blind 6
sketch "Эскиз46" plane through (0, -3, 0) normal (0, -1, 0) x (1, 0, 0)
  circle A0 centre (45, -16.125) radius 21.15 construction
  line L0 (23.85, 5.025) -> (66.15, 5.025) construction
  line L1 (66.15, 5.025) -> (66.15, -37.275) construction
  line L2 (66.15, -37.275) -> (23.85, -37.275) construction
  line L3 (23.85, -37.275) -> (23.85, 5.025) construction
  line L4 (21.85, 7.025) -> (68.15, 7.025)
  line L5 (68.15, 7.025) -> (68.15, -39.275)
  line L6 (68.15, -39.275) -> (21.85, -39.275)
  line L7 (21.85, -39.275) -> (21.85, 7.025)
  point P0 (0, 0)
  dimension "d249" = 2
  dimension "d250" = 2
  dimension "d251" = 2
  dimension "d252" = 2
  constraints: 16 end point, 4 parallel, 4 tangent, 2 horizontal, 2 perpendicular
  measures "d249" distance between parallel lines of L0 L4
  measures "d250" distance between parallel lines of L1 L5
  measures "d251" distance between parallel lines of L6 L2
  measures "d252" distance between parallel lines of L3 L7
extrude "Выдавливание42" add sketch "Эскиз46" against normal blind 2
fillet "Сопряжение21" radius 11.15 6 edges at (21.85, -2, -4.125) (21.85, -2, -28.125) (68.15, -2, -39.275) (68.15, -2, 7.025) (42.175, -1, -28.125) (42.175, -1, -4.125)
fillet "Сопряжение22" radius 5.65 1 edges at (62.5, -1, -16.125)
fillet "Сопряжение23" radius 2 1 edges at (23.85, -3, -16.125)
sketch "Эскиз47" plane through (45, -9, -16.125) normal (0, -1, 0) x (1, 0, 0)
  circle A0 centre (0, 0) radius 18.65 projected
  circle A1 centre (0, 0) radius 18.4
  line L0 (0, 0) -> (18.6484, 0.2441)
  line L1 (18.6484, -0.2441) -> (0, 0)
  line L2 (18.6484, 0.2441) -> (18.6484, -0.2441)
  line L3 (18.6484, -0.2441) -> (18.212, 0)
  line L4 (18.212, 0) -> (18.6484, 0.2441)
  line L5 (18.212, 0) -> (0, 0)
  point P0 (-45, 16.125)
  point P1 (18.3984, 0.2408)
  point P2 (18.3984, -0.2408)
  dimension "d259" = 0.25
  dimension "d260" = 1.5
  dimension "d261" = 0.5
  constraints: 12 end point, 2 point on circle, 1 centre point, 1 coincident, 1 equal length, 1 horizontal
  measures "d259" radial gap between concentric circles of A1 A0
  measures "d260" angle of L1 L0
  measures "d261" distance of L1.start L3.end
extrude "Выдавливание43" add sketch "Эскиз47" against normal up to surface (6 mm away) contours A0 L3 A1 L4 | L4 A1 L0 | L1 A1 L3
fillet "Сопряжение24" radius 0.5 4 edges at (63.6484, -6, -16.3691) (63.6484, -6, -15.8809) (63.3984, -6, -16.3658) (63.3984, -6, -15.8842)
pattern_circular "Круговой массив2" count 12 over 360 about axis through (45, -3, -16.125) along (0, -1, 0) of "Выдавливание43", "Сопряжение24"
fillet "Сопряжение25" radius 0.5 145 edges at (44.4962, -3, 2.4852) (44.8076, -3, 2.3056) (45, -3, 2.275) (45.1924, -3, 2.3056) (45.5038, -3, 2.4852) (49.827, -3, 1.8895) (53.8688, -3, 0.2438) (54.0487, -3, -0.0675) (54.2, -3, -0.1901) (54.3819, -3, -0.2599) (54.7414, -3, -0.26) (58.1875, -3, -2.9375) (60.865, -3, -6.3836) (60.8651, -3, -6.7431) (60.9349, -3, -6.925) (61.0575, -3, -7.0763) (61.3688, -3, -7.2562) (63.0145, -3, -11.298) (63.6102, -3, -15.6212) (63.4306, -3, -15.9326) (63.4, -3, -16.125) (63.4306, -3, -16.3174) (63.6102, -3, -16.6288) (63.0145, -3, -20.952) (61.3688, -3, -24.9938) (61.0575, -3, -25.1737) (60.9349, -3, -25.325) (60.8651, -3, -25.5069) (60.865, -3, -25.8664) (58.1875, -3, -29.3125) (54.7414, -3, -31.99) (54.3819, -3, -31.9901) (54.2, -3, -32.0599) (54.0487, -3, -32.1825) (53.8688, -3, -32.4938) (49.827, -3, -34.1395) (45.5038, -3, -34.7352) (45.1924, -3, -34.5556) (45, -3, -34.525) (44.8076, -3, -34.5556) (44.4962, -3, -34.7352) (40.173, -3, -34.1395) (36.1312, -3, -32.4938) (35.9513, -3, -32.1825) (35.8, -3, -32.0599) (35.6181, -3, -31.9901) (35.2586, -3, -31.99) (31.8125, -3, -29.3125) (29.135, -3, -25.8664) (29.1349, -3, -25.5069) (29.0651, -3, -25.325) (28.9425, -3, -25.1737) (28.6312, -3, -24.9938) (26.9855, -3, -20.952) (26.3898, -3, -16.6288) (26.5694, -3, -16.3174) (26.6, -3, -16.125) (26.5694, -3, -15.9326) (26.3898, -3, -15.6212) (26.9855, -3, -11.298) (28.6312, -3, -7.2562) (28.9425, -3, -7.0763) (29.0651, -3, -6.925) (29.1349, -3, -6.7431) (29.135, -3, -6.3836) (31.8125, -3, -2.9375) (35.2586, -3, -0.26) (35.6181, -3, -0.2599) (35.8, -3, -0.1901) (35.9513, -3, -0.0675) (36.1312, -3, 0.2438) (40.173, -3, 1.8895) (44.4962, -9, 2.4852) (44.8076, -9, 2.3056) (45, -9, 2.275) (45.1924, -9, 2.3056) (45.5038, -9, 2.4852) (49.827, -9, 1.8895) (53.8688, -9, 0.2438) (54.0487, -9, -0.0675) (54.2, -9, -0.1901) (54.3819, -9, -0.2599) (54.7414, -9, -0.26) (58.1875, -9, -2.9375) (60.865, -9, -6.3836) (60.8651, -9, -6.7431) (60.9349, -9, -6.925) (61.0575, -9, -7.0763) (61.3688, -9, -7.2562) (63.0145, -9, -11.298) (63.6102, -9, -15.6212) (63.4306, -9, -15.9326) (63.4, -9, -16.125) (63.4306, -9, -16.3174) (63.6102, -9, -16.6288) (63.0145, -9, -20.952) (61.3688, -9, -24.9938) (61.0575, -9, -25.1737) (60.9349, -9, -25.325) (60.8651, -9, -25.5069) (60.865, -9, -25.8664) (58.1875, -9, -29.3125) (54.7414, -9, -31.99) (54.3819, -9, -31.9901) (54.2, -9, -32.0599) (54.0487, -9, -32.1825) (53.8688, -9, -32.4938) (49.827, -9, -34.1395) (45.5038, -9, -34.7352) (45.1924, -9, -34.5556) (45, -9, -34.525) (44.8076, -9, -34.5556) (44.4962, -9, -34.7352) (40.173, -9, -34.1395) (36.1312, -9, -32.4938) (35.9513, -9, -32.1825) (35.8, -9, -32.0599) (35.6181, -9, -31.9901) (35.2586, -9, -31.99) (31.8125, -9, -29.3125) (29.135, -9, -25.8664) (29.1349, -9, -25.5069) (29.0651, -9, -25.325) (28.9425, -9, -25.1737) (28.6312, -9, -24.9938) (26.9855, -9, -20.952) (26.3898, -9, -16.6288) (26.5694, -9, -16.3174) (26.6, -9, -16.125) (26.5694, -9, -15.9326) (26.3898, -9, -15.6212) (26.9855, -9, -11.298) (28.6312, -9, -7.2562) (28.9425, -9, -7.0763) (29.0651, -9, -6.925) (29.1349, -9, -6.7431) (29.135, -9, -6.3836) (31.8125, -9, -2.9375) (35.2586, -9, -0.26) (35.6181, -9, -0.2599) (35.8, -9, -0.1901) (35.9513, -9, -0.0675) (36.1312, -9, 0.2438) (40.173, -9, 1.8895) (23.85, -9, -16.125)
sketch "Эскиз48" plane through (0, -3, 0) normal (0, -1, 0) x (1, 0, 0)
  circle A0 centre (45, -16.125) radius 21.15 construction
  circle A1 centre (45, -16.125) radius 15
  point P0 (0, 0)
  dimension "d269" = 30
  constraints: 1 centre point, 1 coincident
  measures "d269" diameter of A1
extrude "Выдавливание44" cut sketch "Эскиз48" against normal blind 0.5
fillet "Сопряжение26" radius 1 17 edges at (-15, 52, -28.125) (-15, 52, -4.125) (18.5842, -3, -31.3908) (-40.9, -3, -28.125) (18.5842, -3, -0.8592) (-40.9, -3, -4.125) (-92.5, 24.5, -28.125) (-92.5, 24.5, -4.125) (-92.5, 52, -16.125) (-92.5, -3, -16.125) (62.5, 7.3059, -28.4938) (63.5191, 1.4131, -32.3475) (62.5, 31.075, -28.125) (62.5, 7.3059, -3.7562) (63.5172, 1.4158, 0.0942) (62.5, 31.075, -4.125) (62.5, 52, -16.125)
sketch "Эскиз19" plane through (-15, -3, -32.25) normal (-1, 0, 0) x (0, 0, 1)
  line L0 (32.25, 0) -> (32.25, 54) projected
  line L1 (0, 54) -> (32.25, 54) projected
  line L2 (0, 0) -> (0, 55) projected
  line L3 (32.25, 0) -> (0, 0) projected
  line L4 (32.25, 0) -> (0, 0) projected
  line L5 (2.125, 0) -> (30.125, 0)
  line L6 (30.125, 0) -> (30.125, 47.7)
  line L7 (30.125, 47.7) -> (2.125, 47.7)
  line L8 (2.125, 47.7) -> (2.125, 0)
  line L9 (2.125, 23.85) -> (0, 23.85) construction
  line L10 (0, 0) -> (0, 55) projected
  line L11 (30.125, 23.85) -> (32.25, 23.85) construction
  point P0 (32.25, 3)
  dimension "d108" = 47.7
  dimension "d109" = 28
  constraints: 12 end point, 4 point on line, 2 collinear, 2 horizontal, 2 midpoint, 2 parallel, 1 perpendicular
  measures "d108" distance between parallel lines of L3 L7
  measures "d109" distance between parallel lines of L6 L8
sketch "Эскиз20" plane through (-21, -2, -32.25) normal (-1, 0, 0) x (0, 0, 1)
  line L0 (2.125, 47.7) -> (2.125, 0) projected
  line L1 (2.125, 0) -> (30.125, 0) projected
  line L2 (30.125, 0) -> (30.125, 47.7) projected
  line L3 (30.125, 47.7) -> (2.125, 47.7) projected
  line L4 (30.125, 0) -> (2.125, 47.7) construction
  line L5 (26.125, 43.7) -> (6.125, 43.7)
  line L6 (6.125, 43.7) -> (6.125, 4)
  line L7 (6.125, 4) -> (26.125, 4)
  line L8 (26.125, 4) -> (26.125, 43.7)
  line L9 (26.125, 43.7) -> (6.125, 4) construction
  line L10 (6.125, 43.7) -> (26.125, 4) construction
  point P0 (32.25, 2)
  point P1 (16.125, 23.85)
  dimension "d113" = 4
  dimension "d114" = 4
  constraints: 14 end point, 3 midpoint, 2 parallel, 1 horizontal, 1 perpendicular
  measures "d113" distance between parallel lines of L1 L7
  measures "d114" distance between parallel lines of L0 L6
sketch "Эскиз21" plane through (-21, -2, -32.25) normal (-1, 0, 0) x (0, 0, 1)
  line L0 (26.125, 43.7) -> (6.125, 43.7) construction
  line L1 (6.125, 43.7) -> (6.125, 4) construction
  line L2 (6.125, 4) -> (26.125, 4) construction
  line L3 (26.125, 4) -> (26.125, 43.7) construction
  line L4 (6.125, 4) -> (26.125, 4) construction
  line L5 (26.125, 4) -> (26.125, 43.7) construction
  line L6 (6.125, 4) -> (26.125, 43.7) construction
  line L7 (6.125, 43.7) -> (6.125, 4) construction
  line L8 (26.125, 4) -> (6.125, 43.7) construction
  line L9 (16.125, 4) -> (16.125, 23.85) construction
  circle A0 centre (16.125, 13.8) radius 3.075
  point P0 (32.25, 2)
  dimension "d117" = 9.8
  dimension "d118" = 6.15
  constraints: 6 end point, 2 midpoint, 1 centre point, 1 perpendicular, 1 point on line
  measures "d117" distance from line of L2 A0.centre
  measures "d118" diameter of A0
sketch "Эскиз22" plane through (-21, -2, -32.25) normal (-1, 0, 0) x (0, 0, 1)
  circle A0 centre (16.125, 13.8) radius 3.075 projected
  circle A1 centre (16.125, 13.8) radius 6.5
  point P0 (32.25, 2)
  dimension "d121" = 13
  constraints: 1 centre point, 1 coincident
  measures "d121" diameter of A1